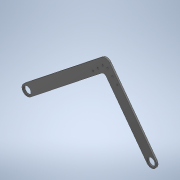
# Autodesk Inventor part: winch_support_mount
Saved by Autodesk Inventor 2020.2 (Build 242310000, 310)
## iProperties
Created: 2020-03-28
Part Number: winch_support_mount
Material: Acetal Resin, Black
Document SubType Name: Modeling
Designer: agmle
Density: 1.425 g/cm^3
Appearance: Smooth - Black
Author: agmle
Autodesk Inventor part; units mm, degrees
ref_plane "YZ Plane" through (0, 0, 0) normal (1, 0, 0) x (0, 1, 0)
ref_plane "XZ Plane" through (0, 0, 0) normal (0, 1, 0) x (-1, 0, 0)
ref_plane "XY Plane" through (0, 0, 0) normal (0, 0, 1) x (1, 0, 0)
sketch "Sketch1" plane through (0, 0, 0) normal (0, 0, 1) x (1, 0, 0)
  line L0 (-245.3259, 0) -> (63.2798, 244.4632) construction
  line L1 (63.2798, 244.4632) -> (245.3259, 0) construction
  line L2 (245.3259, 0) -> (-245.3259, 0) construction
  circle A0 centre (-245.3259, 0) radius 14.7955 construction
  circle A1 centre (245.3259, 0) radius 14.7955 construction
  line L3 (50.1497, 261.0383) -> (-258.4559, 16.5751)
  line L4 (80.2394, 257.0926) -> (262.2855, 12.6295)
  line L5 (-232.1959, -16.5751) -> (49.0756, 206.2352)
  line L6 (67.1475, 203.8654) -> (228.3663, -12.6295)
  arc A2 (80.2394, 257.0926) -> (50.1497, 261.0383) centre (63.2798, 244.4632) ccw
  arc A3 (228.3663, -12.6295) -> (262.2855, 12.6295) centre (245.3259, 0) ccw
  arc A4 (-258.4559, 16.5751) -> (-232.1959, -16.5751) centre (-245.3259, 0) ccw
  arc A5 (67.1475, 203.8654) -> (49.0756, 206.2352) centre (56.9615, 196.2802) ccw
  point P0 (0, 0)
  point P1 (0, 0)
  dimension "d0" = 304.8
  dimension "d1" = 393.7
  dimension "d2" = 490.6518
  dimension "d3" = 29.591
  dimension "d4" = 12.7
  dimension "d14" = 6.35
  constraints: 14 end point, 8 point on circle, 8 tangent, 6 centre point, 6 coincident, 3 parallel, 2 equal radius, 1 horizontal, 1 midpoint
  measures "d0" distance of L0.end L1.end
  measures "d1" distance of L0.start L0.end
  measures "d2" distance of L1.end L0.start
  measures "d3" diameter of A0
  measures "d4" radius of A5
  measures "d14" radial gap between concentric circles of A4 A0
extrude "Frame" add sketch "Sketch1" along normal blind 6
sketch "Sketch2" plane through (0, 0, 6) normal (0, 0, 1) x (1, 0, 0)
  arc A0 (228.3663, -12.6295) -> (262.2855, 12.6295) centre (245.3259, 0) ccw projected
  arc A1 (-258.4559, 16.5751) -> (-232.1959, -16.5751) centre (-245.3259, 0) ccw projected
  point P0 (0, 0)
  point P1 (245.3259, 0)
  point P2 (-245.3259, 0)
  constraints: 2 coincident
hole "Struts" at (245.3259, 0, 6) at (-245.3259, 0, 6) direction (0, 0, -1) diameter 29.591 end through all start extended yes
sketch "Sketch3" plane through (0, 0, 6) normal (0, 0, 1) x (1, 0, 0)
  line L0 (3.112, 193.2757) -> (114.4672, 304.6309) construction
  line L1 (114.4672, 304.6309) -> (123.4475, 295.6506) construction
  line L2 (123.4475, 295.6506) -> (12.0923, 184.2955) construction
  line L3 (12.0923, 184.2955) -> (3.112, 193.2757) construction
  line L4 (114.4672, 184.2955) -> (123.4475, 193.2757) construction
  line L5 (123.4475, 193.2757) -> (12.0923, 304.6309) construction
  line L6 (12.0923, 304.6309) -> (3.112, 295.6506) construction
  line L7 (3.112, 295.6506) -> (114.4672, 184.2955) construction
  circle A0 centre (63.2798, 244.4632) radius 6.35 construction
  line L8 (3.112, 295.6506) -> (3.112, 193.2757) construction
  arc A1 (80.2394, 257.0926) -> (50.1497, 261.0383) centre (63.2798, 244.4632) ccw construction
  line L9 (58.7896, 239.973) -> (7.6022, 188.7856) construction
  line L10 (67.7699, 239.973) -> (118.9573, 188.7856) construction
  line L11 (53.7548, 234.9382) -> (72.8048, 234.9382) construction
  line L12 (91.8548, 215.8882) -> (34.7048, 215.8882) construction
  line L13 (110.9048, 196.8382) -> (15.6548, 196.8382) construction
  line L14 (63.2798, 196.8382) -> (63.2798, 215.8882) construction
  line L15 (63.2798, 215.8882) -> (63.2798, 234.9382) construction
  point P0 (0, 0)
  point P1 (58.7896, 248.9533)
  dimension "d15" = 12.7
  dimension "d16" = 157.48
  dimension "d17" = 19.05
  dimension "d18" = 3.175
  constraints: 32 end point, 8 midpoint, 7 equal length, 7 point on line, 3 perpendicular, 3 point on circle, 3 tangent, 2 parallel, 1 centre point, 1 collinear, 1 concentric, 1 horizontal, 1 vertical
  measures "d15" distance of L5.end L6.end
  measures "d16" distance of L4.end L5.end
  measures "d17" distance of L14.end L15.end
  measures "d18" distance edge to line of A0 L11
hole "Hole2" at (15.6548, 196.8382, 6) at (34.7048, 215.8882, 6) at (53.7548, 234.9382, 6) at (72.8048, 234.9382, 6) at (91.8548, 215.8882, 6) at (110.9048, 196.8382, 6) direction (0, 0, -1) diameter 3.4036 end through all start extended yes countersink diameter 6.2992 countersink angle 90 clearance for "Flat Head Machine Screw" size "M3" standard "Ansi Metric M Profile"
body "Solid1"
